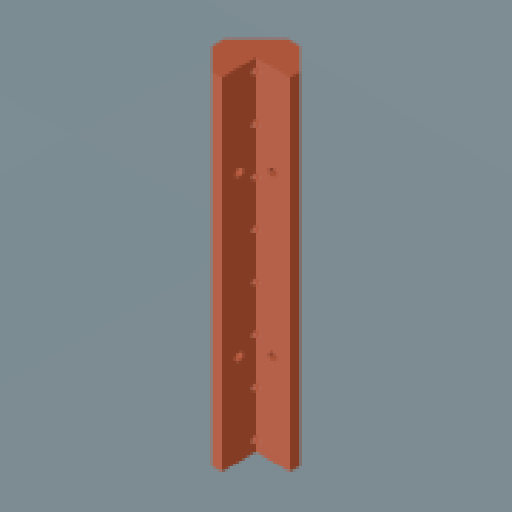
# Autodesk Inventor part: Corner Z Brace
Saved by Autodesk Inventor 2023.2 (Build 272271000, 271)
## iProperties
Created: 2023-02-15
Part Number: Corner Z Brace
Material: ABS Plastic
Document SubType Name: Modeling
Designer: remop
Density: 1.06 g/cm^3
Appearance: Smooth - Light Orange
Author: remop
Autodesk Inventor part; units mm, degrees
ref_plane "YZ Plane" through (0, 0, 0) normal (1, 0, 0) x (0, 1, 0)
ref_plane "XZ Plane" through (0, 0, 0) normal (0, 1, 0) x (-1, 0, 0)
ref_plane "XY Plane" through (0, 0, 0) normal (0, 0, 1) x (1, 0, 0)
sketch "Sketch1" plane through (0, 0, 0) normal (0, 1, 0) x (-1, 0, 0)
  line L0 (0, 0) -> (0, 15)
  line L1 (0, 15) -> (14.1421, 15)
  line L2 (14.1421, 15) -> (14.1421, 0)
  line L3 (14.1421, 0) -> (0, -14.1421)
  line L4 (0, -14.1421) -> (-15, -14.1421)
  line L5 (-15, -14.1421) -> (-15, 0)
  line L6 (-15, 0) -> (0, 0)
  dimension "d0" = 15
  dimension "d1" = 10
  constraints: 14 end point, 7 perpendicular, 1 parallel, 1 point on line, 1 vertical
  measures "d0" distance of L0.start L0.end
  measures "d1" distance from line of L0.start L3
extrude "Extrusion1" add sketch "Sketch1" along normal blind 150
chamfer "Chamfer1" distance 10 angle 45 2 edges at (-14.1421, 75, 15) (15, 75, -14.1421)
sketch "Sketch2" plane through (-14.1421, 0, 0) normal (-1, 0, 0) x (0, 0, 1)
  line L0 (15, 150) -> (5, 150) projected
  line L1 (5, 150) -> (5, 0) projected
  line L2 (5, 0) -> (15, 0) projected
  line L3 (15, 0) -> (15, 150) projected
  line L4 (5, 150) -> (5, 0) projected
  line L5 (0, 150) -> (5, 150) projected
  line L6 (0, 0) -> (0, 150) projected
  line L7 (0, 0) -> (5, 0) projected
  point P0 (0, 0)
  point P1 (7.5, 40)
  point P2 (7.5, 110)
  dimension "d7" = 7.5
  dimension "d8" = 40
  dimension "d9" = 40
  constraints: 1 vertical alignment
  measures "d7" distance from line of L3 point (7.5, 40)
  measures "d8" distance from line of L2 point (7.5, 40)
  measures "d9" distance from line of L0 point (7.5, 110)
hole "Hole1" at (-14.1421, 40, 7.5) at (-14.1421, 110, 7.5) direction (1, 0, 0) diameter 3.6 end through all counterbore diameter 6.5 counterbore depth 10 clearance for "Socket Head Cap Screw ISO 4762" size "M3" standard "ISO"
sketch "Sketch3" plane through (0, 0, -14.1421) normal (0, 0, -1) x (-1, 0, 0)
  line L0 (-5, 150) -> (-15, 150) projected
  line L1 (-15, 150) -> (-15, 0) projected
  line L2 (-15, 0) -> (-5, 0) projected
  line L3 (-5, 0) -> (-5, 150) projected
  line L4 (-5, 0) -> (-5, 150) projected
  line L5 (-5, 0) -> (0, 0) projected
  line L6 (0, 0) -> (0, 150) projected
  line L7 (-5, 150) -> (0, 150) projected
  point P0 (-7.5, 40)
  point P1 (-7.5, 110)
  dimension "d17" = 40
  dimension "d18" = 40
  dimension "d26" = 7.5
  constraints: 1 vertical alignment
  measures "d17" distance from line of L2 point (-7.5, 40)
  measures "d18" distance from line of L0 point (-7.5, 110)
  measures "d26" distance from line of L1 point (-7.5, 40)
hole "Hole2" at (7.5, 40, -14.1421) at (7.5, 110, -14.1421) direction (0, 0, 1) diameter 3.6 end through all counterbore diameter 6.5 counterbore depth 10
sketch "Sketch4" plane through (-14.1421, 0, 0) normal (-0.7071, 0, -0.7071) x (-0.7071, 0, 0.7071)
  circle A0 centre (-10, 25) radius 3 projected
  circle A1 centre (-10, 65) radius 3 projected
  circle A2 centre (-10, 105) radius 3 projected
  circle A3 centre (-10, 145) radius 3 projected
  circle A4 centre (-10, 185) radius 3 projected
  circle A5 centre (-10, 225) radius 3 projected
  circle A6 centre (-10, 265) radius 3 projected
  circle A7 centre (-10, 285) radius 3 projected
  circle A8 centre (-10, 245) radius 3 projected
  circle A9 centre (-10, 205) radius 3 projected
  circle A10 centre (-10, 165) radius 3 projected
  circle A11 centre (-10, 125) radius 3 projected
  circle A12 centre (-10, 85) radius 3 projected
  circle A13 centre (-10, 45) radius 3 projected
  circle A14 centre (-10, 5) radius 3 projected
  line L0 (-5.5, 290) -> (-14.5, 290) projected
  line L1 (-14.5, 290) -> (-14.5, -60) projected
  line L2 (-5.5, -60) -> (-14.5, -60) projected
  line L3 (-5.5, 290) -> (-5.5, -60) projected
  circle A15 centre (-10, -55) radius 3 projected
  circle A16 centre (-10, -15) radius 3 projected
  circle A17 centre (-10, -35) radius 3 projected
  point P0 (-10, 0)
hole "Hole3" at (-7.0711, 165, -7.0711) at (-7.0711, 145, -7.0711) at (-7.0711, 125, -7.0711) at (-7.0711, 105, -7.0711) at (-7.0711, 85, -7.0711) at (-7.0711, 65, -7.0711) at (-7.0711, 45, -7.0711) at (-7.0711, 25, -7.0711) at (-7.0711, 5, -7.0711) direction (0.7071, 0, 0.7071) diameter 2.8 end through all
equation "\"d9\" = d8"
equation "\"d18\" = d17"
body "Solid1"
